VIHALS Motor Top Wire Holder (Autodesk Fusion 360 design; units mm, degrees)
Autodesk Fusion 360 part; units mm, degrees
sketch "Sketch1" plane through (0, 0, 0) normal (0, 0, 1) x (1, 0, 0)
  line L0 (-12.5, 10) -> (12.5, 10)
  line L1 (12.5, 10) -> (12.5, -10)
  line L2 (12.5, -10) -> (-12.5, -10)
  line L3 (-12.5, -10) -> (-12.5, 10)
  dimension "d1" = 20
  dimension "d2" = 25
  dimension "d3" = 12.5
  dimension "d4" = 10
  constraint horizontal L0
  constraint vertical L1
  constraint horizontal L2
  constraint vertical L3
  measures "d1" distance of L0 L2
  measures "d2" distance of L1 L3
  measures "d3" distance of origin L3
  measures "d4" distance of origin L2
extrude "Extrude1" add sketch "Sketch1" along normal blind 3
sketch "Sketch2" plane through (0, 0, 3) normal (0, 0, 1) x (-1, 0, 0)
  line L0 (12.5, 10) -> (-12.5, 10)
  line L1 (-12.5, 10) -> (-12.5, -10)
  line L2 (-12.5, -10) -> (12.5, -10)
  line L3 (12.5, -10) -> (12.5, 10)
  line L4 (27, 1.25) -> (27, -1.25)
  line L5 (12.5, 10) -> (12.5, -10)
  circle A0 centre (15.5, 1.25) radius 5
  circle A1 centre (15.5, -1.25) radius 5
  line L6 (27, -1.25) -> (15.5, -1.25)
  circle A2 centre (15.5, -1.25) radius 3
  line L7 (15.5, -1.25) -> (12.5, -1.25)
  circle A3 centre (15.5, 1.25) radius 3
  line L8 (15.5, 1.25) -> (12.5, 1.25)
  line L9 (15.5, 1.25) -> (27, 1.25)
  point P0 (10.5, 0)
  dimension "d7" = 10
  dimension "d8" = 10
  dimension "d10" = 2.5
  dimension "d12" = 6
  dimension "d13" = 6
  dimension "d14" = 2
  constraint concentric A0 A3
  constraint concentric A1 A2
  constraint coincident A0.centre A3.centre
  constraint coincident L8.end L5
  constraint perpendicular L5 L8
  constraint coincident A1.centre L6.end
  constraint coincident L7.end L5
  constraint perpendicular L5 L7
  constraint parallel L7 L9
  constraint perpendicular L4 L9
  constraint perpendicular L4 L6
  constraint horizontal origin P0
  constraint coincident L2.end L3.start
  measures "d7" diameter of A0
  measures "d8" diameter of A1
  measures "d10" distance of A0.centre A1.centre
  measures "d12" diameter of A3
  measures "d13" diameter of A2
  measures "d14" distance of P0 L5
extrude "Extrude2" add sketch "Sketch2" against normal blind 3 contours L3 L5 A0 A1 A3 L9 | L3 L5 A1 A3 | A1 A3 L9 | L3 L5 A0 A1 L6 A2 | L3 L5 A0 A2 | A0 L6 A2
fillet "Fillet1" radius 1 2 edges at (-20.5, -1.25, 1.5) (-20.5, 1.25, 1.5)
fillet "Fillet1" radius 50 2 edges at (-12.5, 5.25, 1.5) (-12.5, -5.25, 1.5)
sketch "Sketch3" plane through (0, 0, 3) normal (0, 0, 1) x (-1, 0, 0)
  arc A0 (20.3412, -2.5) -> (19.373, -1.25) centre (19.373, -2.25) ccw
  line L0 (19.373, -1.25) -> (18.5, -1.25)
  arc A1 (12.5, -1.25) -> (18.5, -1.25) centre (15.5, -1.25) ccw
  line L1 (12.5, -1.25) -> (12.5, 1.25)
  arc A2 (18.5, 1.25) -> (12.5, 1.25) centre (15.5, 1.25) ccw
  line L2 (18.5, 1.25) -> (19.373, 1.25)
  arc A3 (19.373, 1.25) -> (20.3412, 2.5) centre (19.373, 2.25) ccw
  arc A4 (20.3412, 2.5) -> (18.3105, 5.3854) centre (15.5, 1.25) ccw
  arc A5 (12.5, 10) -> (18.3105, 5.3854) centre (46.4154, 46.7389) ccw
  line L3 (12.5, 10) -> (-12.5, 10)
  line L4 (-12.5, 10) -> (-12.5, -10)
  line L5 (-12.5, -10) -> (12.5, -10)
  arc A6 (18.3105, -5.3854) -> (12.5, -10) centre (46.4154, -46.7389) ccw
  arc A7 (18.3105, -5.3854) -> (20.3412, -2.5) centre (15.5, -1.25) ccw
  point P0 (3, -4)
  point P1 (-7, 4)
  dimension "d32" = 5.5
  dimension "d33" = 4
  dimension "d34" = 4
  dimension "d41" = 10
  measures "d32" distance of L4 P1
  measures "d33" vertical distance of origin P1
  measures "d34" vertical distance of origin P0
  measures "d41" horizontal distance of P0 P1
hole "Hole2" at (-3, 4, 3) at (7, -4, 3) direction (0, 0, -1) diameter 3.797 depth 6 tip angle 118 countersink diameter 7.087 countersink angle 100
